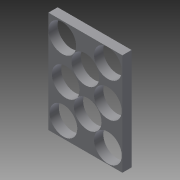
# Autodesk Inventor part: 5.1 Q6
Saved by Autodesk Inventor 2015 (Build 190159000, 159)
## iProperties
Created: 2017-11-28
Part Number: 5.1 Q6
Material: Generic
Document SubType Name: Modeling
Designer: Administrator
Density: 1 g/cm^3
Appearance: Default
Author: Administrator
Autodesk Inventor part; units mm, degrees
ref_plane "YZ Plane" through (0, 0, 0) normal (1, 0, 0) x (0, 1, 0)
ref_plane "XZ Plane" through (0, 0, 0) normal (0, 1, 0) x (-1, 0, 0)
ref_plane "XY Plane" through (0, 0, 0) normal (0, 0, 1) x (1, 0, 0)
sketch "Sketch1" plane through (0, 0, 0) normal (0, 0, 1) x (1, 0, 0)
  line L0 (0, 0) -> (0, 279.4)
  line L1 (0, 279.4) -> (203.2, 279.4)
  line L2 (203.2, 279.4) -> (203.2, 0)
  line L3 (203.2, 0) -> (0, 0)
  circle A0 centre (101.6, 195.2625) radius 38.1
  circle A1 centre (163.5125, 39.6875) radius 38.1
  circle A2 centre (41.275, 42.8625) radius 38.1
  circle A3 centre (107.95, 92.075) radius 38.1
  circle A4 centre (163.5125, 146.05) radius 38.1
  circle A5 centre (47.625, 138.1125) radius 38.1
  circle A6 centre (38.1, 238.125) radius 38.1
  circle A7 centre (163.5125, 241.3) radius 38.1
  dimension "d0" = 203.2
  dimension "d1" = 279.4
  dimension "d2" = 76.2
  dimension "d3" = 76.2
  dimension "d4" = 76.2
  dimension "d5" = 76.2
  dimension "d6" = 76.2
  dimension "d7" = 76.2
  dimension "d8" = 76.2
  dimension "d9" = 76.2
  constraints: 8 centre point, 8 end point, 3 perpendicular, 1 vertical
  measures "d0" distance of L0.end L1.end
  measures "d1" distance of L0.start L0.end
  measures "d2" diameter of A0
  measures "d3" diameter of A1
  measures "d4" diameter of A2
  measures "d5" diameter of A3
  measures "d6" diameter of A4
  measures "d7" diameter of A5
  measures "d8" diameter of A6
  measures "d9" diameter of A7
extrude "Extrusion1" add sketch "Sketch1" along normal blind 25.4
body "Solid1"
